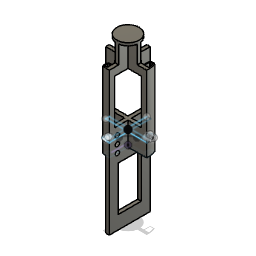
Sensor Holder -Fusion360 (Autodesk Fusion 360 design; units mm, degrees)
Autodesk Fusion 360 part; units mm, degrees
note: some values were not read from the file. Set by a fixed rule: which sketch regions a step uses.
sketch "Sketch1" plane through (0, 0, 0) normal (0, 1, 0) x (1, 0, 0)
  line L0 (2, 2) -> (2, 22.9129)
  line L1 (-2, 2) -> (-2, 22.9129)
  line L2 (-2, -2) -> (-22.9129, -2)
  line L3 (-2, 2) -> (-22.9129, 2)
  line L4 (2, -2) -> (2, -22.9129)
  line L5 (-2, 2) -> (-2, 22.9129)
  line L6 (2, -2) -> (22.9129, -2)
  line L7 (-2, -2) -> (-22.9129, -2)
  line L8 (2, 2) -> (15.8617, 2)
  arc A0 (21.3471, 2.5595) -> (20.9546, 4.8119) centre (0, 0) ccw
  arc A1 (20.8507, 2) -> (21.3471, 2.5595) centre (20.8507, 2.5) ccw
  arc A2 (16.8617, 2.5) -> (17.3617, 2) centre (17.3617, 2.5) ccw
  line L9 (-2, 2) -> (2, -2) construction
  line L10 (-6.2, -22.1486) -> (-6.2, -20.8617)
  line L11 (-6.2, -20.8617) -> (-6.2, -17.8617)
  arc A3 (-4.2, -15.8617) -> (-6.2, -17.8617) centre (-4.2, -17.8617) ccw
  line L12 (-4.2, -15.8617) -> (-2, -15.8617)
  line L13 (-4.2, -16.8617) -> (-2.5, -16.8617)
  arc A4 (-2, -17.3617) -> (-2.5, -16.8617) centre (-2.5, -17.3617) ccw
  arc A5 (-2.5595, -21.3471) -> (-2, -20.8507) centre (-2.5, -20.8507) ccw
  arc A6 (-4.8119, -20.9546) -> (-2.5595, -21.3471) centre (0, 0) ccw
  arc A7 (-5.2, -20.4673) -> (-4.8119, -20.9546) centre (-4.7, -20.4673) ccw
  line L14 (-5.2, -20.4673) -> (-5.2, -17.8617)
  arc A8 (-4.2, -16.8617) -> (-5.2, -17.8617) centre (-4.2, -17.8617) ccw
  line L15 (-2, -2) -> (-2, -15.8617)
  line L16 (-2, -17.3617) -> (-2, -20.8507)
  line L17 (17.3617, 2) -> (17.6582, 2)
  line L18 (17.6582, 2) -> (20.8507, 2)
  arc A9 (2, 22.9129) -> (-2, 22.9129) centre (0, 0) ccw
  arc A10 (-22.9129, 2) -> (-22.9129, -2) centre (0, 0) ccw
  arc A11 (-6.2, -22.1486) -> (2, -22.9129) centre (0, 0) ccw
  arc A12 (22.9129, -2) -> (22.1486, 6.2) centre (0, 0) ccw
  line L19 (19.9562, 8) -> (17.3617, 8)
  line L20 (16.8617, 2.5) -> (16.8617, 7.5)
  arc A13 (17.3617, 8) -> (16.8617, 7.5) centre (17.3617, 7.5) ccw
  line L21 (19.5256, 9) -> (17.3617, 9)
  arc A14 (17.3617, 9) -> (15.8617, 7.5) centre (17.3617, 7.5) ccw
  line L22 (15.8617, 2.5) -> (15.8617, 7.5)
  arc A15 (21.3471, 2.5595) -> (19.9562, 8) centre (0, 0) ccw
  line L23 (19.5256, 9) -> (21.166, 9)
  arc A16 (22.9129, -2) -> (21.166, 9) centre (0, 0) ccw
  arc A17 (-6.2, -22.1486) -> (2, -22.9129) centre (0, 0) ccw
  arc A18 (2, 22.9129) -> (-2, 22.9129) centre (0, 0) ccw
  arc A19 (-22.9129, 2) -> (-22.9129, -2) centre (0, 0) ccw
  line L24 (15.8617, 2.5) -> (15.8617, 2)
  point P0 (20.8617, 5.2)
  point P1 (16.8617, 5.2)
  dimension "d1" = 46
  dimension "d21" = 4
  dimension "d25" = 0.5
  dimension "d26" = 0.5
  dimension "d34" = 0.5
  constraint coincident A0.centre A6.centre
  constraint coincident P0 A0
  constraint tangent A0 A1
  constraint collinear L15 L16
  constraint tangent A1 L18
  constraint concentric A9 A10
  constraint concentric A10 A11
  constraint concentric A11 A12
  constraint coincident L6.end A18
  constraint tangent A2 L20
  constraint perpendicular L19 L20
  constraint tangent L20 A13
  constraint tangent L19 A13
  constraint parallel L19 L21
  constraint concentric A13 A14
  constraint parallel L20 L22
  constraint tangent L21 A14
  constraint tangent A14 L22
  constraint parallel L21 L23
  constraint concentric A16 A18
  constraint concentric A17 A18
  constraint concentric A18 A19
  constraint perpendicular L8 L24
  measures "d1" diameter of A9
  measures "d21" distance of P0 P1
  measures "d25" radius of A1
  measures "d26" radius of A2
  measures "d34" radius of A13
sketch "Sketch2" plane through (0, 0, 0) normal (0, 0, 1) x (1, 0, 0)
  line L0 (0, 0) -> (0, 86.0013) construction
  line L1 (-10.6, 11.1415) -> (10.6, 11.1415)
  line L2 (10.6, 11.1415) -> (10.6, 61.3415)
  line L3 (10.6, 61.3415) -> (-10.6, 61.3415)
  line L4 (-10.6, 61.3415) -> (-10.6, 11.1415)
  line L5 (0, 11.1415) -> (0, 0)
  dimension "d2" = 21.2
  dimension "d3" = 50.2
  constraint coincident L0.start L5.end
  constraint vertical L0
  constraint horizontal L1
  constraint vertical L2
  constraint horizontal L3
  constraint vertical L4
  constraint midpoint L1 L5.start
  constraint perpendicular L1 L5
  measures "d2" distance of L1.start L1.end
  measures "d3" distance of L1.start L3.end
extrude "Extrude1" add sketch "Sketch1" along normal blind 70 makes body 1
extrude "Extrude2" add sketch "Sketch2" along normal blind 35 and the other way blind 35 separate body makes body 2
sketch "Sketch3" plane through (0, 0, 0) normal (1, 0, 0) x (0, 0, -1)
move_body "Move1" bodies 2 to x (0.707107, 0, -0.707107) y (0, 1, 0) z (0.707107, 0, 0.707107) at (0, 0, 0)
combine "Combine1" operation cut target body 1 tool bodies 2
sketch "Sketch4" plane through (0, 70, 0) normal (0, 1, 0) x (-1, 0, 0)
  arc A0 (-12.339, 2) -> (-12.339, -2) centre (0, 0) ccw
  arc A1 (2, 12.339) -> (-2, 12.339) centre (0, 0) ccw
  arc A2 (-2, -12.339) -> (2, -12.339) centre (0, 0) ccw
  arc A3 (12.339, -2) -> (12.339, 2) centre (0, 0) ccw
  line L0 (2, -2) -> (12.339, -2)
  line L1 (2, 2) -> (12.339, 2)
  line L2 (2, 2) -> (2, 12.339)
  line L3 (-2, 2) -> (-2, 12.339)
  line L4 (-2, 2) -> (-12.339, 2)
  line L5 (-2, -2) -> (-12.339, -2)
  line L6 (-2, -2) -> (-2, -12.339)
  line L7 (2, -2) -> (2, -12.339)
  dimension "d27" = 25
  constraint concentric A0 A2
  constraint concentric A1 A2
  constraint concentric A2 A3
  measures "d27" diameter of A2
extrude "Extrude3" add sketch "Sketch4" along normal blind 20 bodies 1
sketch "Sketch5" plane through (0, 90, 0) normal (0, 1, 0) x (-1, 0, 0)
  arc A0 (12.339, -2) -> (12.339, 2) centre (0, 0) ccw
  line L0 (12.339, 2) -> (2, 2)
  line L1 (2, 2) -> (2, 12.339)
  arc A1 (2, 12.339) -> (-2, 12.339) centre (0, 0) ccw
  line L2 (-2, 12.339) -> (-2, 2)
  line L3 (-2, 2) -> (-12.339, 2)
  arc A2 (-12.339, 2) -> (-12.339, -2) centre (0, 0) ccw
  line L4 (-12.339, -2) -> (-2, -2)
  line L5 (-2, -2) -> (-2, -12.339)
  arc A3 (-2, -12.339) -> (2, -12.339) centre (0, 0) ccw
  line L6 (2, -12.339) -> (2, -2)
  line L7 (2, -2) -> (12.339, -2)
  circle A4 centre (0, 0) radius 12.5
  constraint concentric A0 A4
  constraint coincident L5.end A4
extrude "Extrude4" add sketch "Sketch5" along normal blind 3 bodies 1
extrude "Extrude5" add sketch "Sketch1" against normal blind 15 bodies 1
sketch "Sketch6" plane through (0, -15, 0) normal (0, -1, 0) x (1, 0, 0)
  arc A0 (17.3617, -2) -> (16.8617, -2.5) centre (17.3617, -2.5) ccw
  line L0 (17.3617, -2) -> (20.8507, -2)
  arc A1 (21.3471, -2.5595) -> (20.8507, -2) centre (20.8507, -2.5) ccw
  arc A2 (19.9562, -8) -> (21.3471, -2.5595) centre (0, 0) ccw
  line L1 (19.9562, -8) -> (17.3617, -8)
  arc A3 (16.8617, -7.5) -> (17.3617, -8) centre (17.3617, -7.5) ccw
  line L2 (16.8617, -7.5) -> (16.8617, -2.5)
  arc A4 (-5.2, 17.8617) -> (-4.2, 16.8617) centre (-4.2, 17.8617) ccw
  line L3 (-5.2, 17.8617) -> (-5.2, 20.4673)
  arc A5 (-4.8119, 20.9546) -> (-5.2, 20.4673) centre (-4.7, 20.4673) ccw
  arc A6 (-2.5595, 21.3471) -> (-4.8119, 20.9546) centre (0, 0) ccw
  arc A7 (-2, 20.8507) -> (-2.5595, 21.3471) centre (-2.5, 20.8507) ccw
  line L4 (-2, 20.8507) -> (-2, 17.3617)
  arc A8 (-2.5, 16.8617) -> (-2, 17.3617) centre (-2.5, 17.3617) ccw
  line L5 (-2.5, 16.8617) -> (-4.2, 16.8617)
  line L6 (17.3617, -9) -> (21.166, -9)
  arc A9 (21.166, -9) -> (22.9129, 2) centre (0, 0) ccw
  line L7 (22.9129, 2) -> (2, 2)
  line L8 (2, 2) -> (2, 22.9129)
  arc A10 (2, 22.9129) -> (-6.2, 22.1486) centre (0, 0) ccw
  line L9 (-6.2, 22.1486) -> (-6.2, 17.8617)
  arc A11 (-6.2, 17.8617) -> (-4.2, 15.8617) centre (-4.2, 17.8617) ccw
  line L10 (-4.2, 15.8617) -> (-2, 15.8617)
  line L11 (-2, 2) -> (-22.9129, 2)
  arc A12 (-22.9129, 2) -> (-22.9129, -2) centre (0, 0) ccw
  line L12 (-22.9129, -2) -> (-2, -2)
  line L13 (-2, -2) -> (-2, -22.9129)
  arc A13 (-2, -22.9129) -> (2, -22.9129) centre (0, 0) ccw
  line L14 (2, -22.9129) -> (2, -2)
  line L15 (2, -2) -> (15.8617, -2)
  line L16 (15.8617, -2) -> (15.8617, -7.5)
  arc A14 (15.8617, -7.5) -> (17.3617, -9) centre (17.3617, -7.5) ccw
  arc A15 (-12.339, -2) -> (-2, -12.339) centre (0, 0) ccw
  line L17 (-2, 15.8617) -> (-2, 2)
  dimension "d38" = 25
  constraint coincident A2.centre A6.centre
  constraint coincident L12 A15.start
  constraint coincident L13 A15.end
  measures "d38" diameter of A15
extrude "Extrude7" add sketch "Sketch6" against normal blind 1.5 contours L12 L13 A15 bodies 1
sketch "Sketch7" plane through (0, -15, 0) normal (0, -1, 0) x (1, 0, 0)
  arc A0 (2, 22.9129) -> (-6.2, 22.1486) centre (0, 0) ccw
  line L0 (2, 2) -> (2, 22.9129)
  line L1 (-2, 2) -> (-2, 15.8617)
  line L2 (-2, -2) -> (-2, -22.9129)
  line L3 (2, -2) -> (2, -22.9129)
  arc A1 (-2, -22.9129) -> (2, -22.9129) centre (0, 0) ccw
  line L4 (-2, 2) -> (-2, -2)
  line L5 (2, 2) -> (2, -2)
  line L6 (-2, 15.8617) -> (-2.1345, 22.9007)
  line L7 (-2, 15.8617) -> (-2, 2)
  line L8 (-2, -2) -> (-2, -22.9129)
  line L9 (2, -22.9129) -> (2, -2)
  line L10 (2, 2) -> (2, 22.9129)
  arc A2 (2, 22.9129) -> (-2.1345, 22.9007) centre (0, 0) ccw
  arc A3 (-2, -22.9129) -> (2, -22.9129) centre (0, 0) ccw
  constraint coincident L1.start L4.start
  constraint coincident L2.start L4.end
  constraint coincident L0.start L5.start
  constraint coincident L3.start L5.end
  constraint coincident L1.end L6.start
  constraint midpoint A0 L6.end
  constraint coincident L2.end A1.start
  constraint coincident L3.end A1.end
  constraint coincident A0.start L0.end
  constraint coincident A0.centre A1.centre
  constraint concentric A2 A3
extrude "Extrude8" add sketch "Sketch7" along normal blind 75 bodies 1
sketch "Sketch8" plane through (2, 0, 0) normal (1, 0, 0) x (0, 0, -1)
  line L0 (12.9907, 11.1415) -> (2, 11.1415)
  line L1 (2, 11.1415) -> (2, -15)
  line L2 (2, -15) -> (-2, -15)
  line L3 (-2, -15) -> (-2, 11.1415)
  line L4 (-2, 11.1415) -> (-16.9907, 11.1415)
  line L5 (-16.9907, 11.1415) -> (-16.9907, 61.3415)
  line L6 (-16.9907, 61.3415) -> (-2, 61.3415)
  line L7 (-2, 61.3415) -> (-2, 90)
  line L8 (-2, 90) -> (-12.339, 90)
  line L9 (-12.339, 90) -> (-12.339, 70)
  line L10 (-12.339, 70) -> (-22.9129, 70)
  line L11 (-22.9129, 70) -> (-22.9129, -90)
  line L12 (-22.9129, -90) -> (22.9129, -90)
  line L13 (22.9129, -90) -> (22.9129, 70)
  line L14 (22.9129, 70) -> (12.339, 70)
  line L15 (12.339, 70) -> (12.339, 90)
  line L16 (12.339, 90) -> (2, 90)
  line L17 (2, 90) -> (2, 61.3415)
  line L18 (2, 61.3415) -> (12.9907, 61.3415)
  line L19 (12.9907, 61.3415) -> (12.9907, 11.1415)
  line L20 (22.9129, -15) -> (-22.9129, -15) construction
  line L21 (0, -15) -> (0, -25) construction
  line L22 (0, -25) -> (0, -75) construction
  line L23 (0, -25) -> (13, -25) construction
  line L24 (0, -75) -> (-13, -75) construction
  line L25 (13, -25) -> (-13, -25)
  line L26 (-13, -25) -> (-13, -75)
  line L27 (-13, -75) -> (13, -75)
  line L28 (13, -75) -> (13, -25)
  line L29 (22.9129, -6.3333) -> (-22.9129, -6.3333) construction
  line L30 (22.9129, 2.3333) -> (-22.9129, 2.3333) construction
  line L31 (-13.9129, 70) -> (-13.9129, -90) construction
  line L32 (15.9129, -90) -> (15.9129, 70) construction
  circle A0 centre (-13.9129, 2.3333) radius 2.5
  circle A1 centre (-13.9129, -15) radius 2.5
  circle A2 centre (15.9129, 2.3333) radius 2.5
  circle A3 centre (15.9129, -6.3333) radius 2.5
  circle A4 centre (15.9129, -15) radius 2.5
  circle A5 centre (-13.9129, -6.3333) radius 2.5
  point P0 (2, -15)
  dimension "d45" = 10
  dimension "d46" = 50
  dimension "d47" = 13
  dimension "d48" = 13
  dimension "d49" = 8.6667
  dimension "d50" = 17.3333
  dimension "d51" = -9
  dimension "d52" = -7
  dimension "d53" = 5
  dimension "d54" = 5
  dimension "d55" = 5
  dimension "d56" = 5
  dimension "d57" = 5
  dimension "d58" = 5
  constraint coincident L13 L20.start
  constraint coincident L11 L20.end
  constraint perpendicular L11 L20
  constraint midpoint L2 L21.start
  constraint perpendicular L2 L21
  constraint parallel L21 L22
  constraint perpendicular L22 L23
  constraint perpendicular L22 L24
  constraint horizontal L25
  constraint vertical L26
  constraint horizontal L27
  constraint vertical L28
  constraint coincident L31 A0.centre
  constraint coincident L30 A0.centre
  constraint coincident L31 A1.centre
  constraint coincident L20 A1.centre
  constraint coincident L30 A2.centre
  constraint coincident L32 A2.centre
  constraint coincident L32 A3.centre
  constraint coincident L29 A3.centre
  constraint coincident L20 A4.centre
  constraint coincident L32 A4.centre
  constraint coincident L29 A5.centre
  constraint coincident L31 A5.centre
  measures "d45" distance of L21.start L21.end
  measures "d46" distance of L21.end L22.end
  measures "d47" distance of L21.end L23.end
  measures "d48" distance of L22.end L24.end
  measures "d53" diameter of A0
  measures "d54" diameter of A1
  measures "d55" diameter of A2
  measures "d56" diameter of A3
  measures "d57" diameter of A4
  measures "d58" diameter of A5
extrude "Extrude9" cut sketch "Sketch8" against normal up to surface (4 mm away) contours L25 L26 L27 L28 | A0 | A1 | A2 | A3 | A4 | A5 bodies 1
equation "d47 = ( 26 / 2 ) * 1 mm"
equation "d48 = ( 26 / 2 ) * 1 mm"
equation "d49 = ( 26 / 3 ) * 1 mm"
equation "d50 = ( 2 * 26 / 3 ) * 1 mm"
